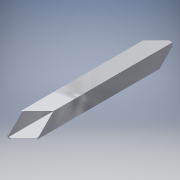
# Autodesk Inventor part: vertical support
Saved by Autodesk Inventor 2016 (Build 200138000, 138)
## iProperties
Created: 2016-02-02
Part Number: vertical support
Material: Aluminum 6061
Document SubType Name: Modeling
Designer: gus
Density: 2.7 g/cm^3
Appearance: Aluminum - Flat
Mass: 93.3295 g
Surface Area: 438.507 cm^2
Volume: 34.5665 cm^3
Author: gus
Autodesk Inventor part; units mm, degrees
ref_plane "YZ Plane" through (0, 0, 0) normal (1, 0, 0) x (0, 1, 0)
ref_plane "XZ Plane" through (0, 0, 0) normal (0, 1, 0) x (-1, 0, 0)
ref_plane "XY Plane" through (0, 0, 0) normal (0, 0, 1) x (1, 0, 0)
sketch "Sketch1" plane through (0, 0, 0) normal (0, 0, 1) x (1, 0, 0)
  line L0 (0, 0) -> (25.4, 0)
  line L1 (25.4, 0) -> (25.4, -25.4)
  line L2 (25.4, -25.4) -> (0, -25.4)
  line L3 (0, -25.4) -> (0, 0)
  line L4 (1.5875, -23.8125) -> (23.8125, -23.8125)
  line L5 (23.8125, -23.8125) -> (23.8125, -1.5875)
  line L6 (23.8125, -1.5875) -> (1.5875, -1.5875)
  line L7 (1.5875, -1.5875) -> (1.5875, -23.8125)
  dimension "d0" = 25.4
  dimension "d1" = 25.4
  dimension "d2" = 1.5875
  constraints: 16 end point, 4 parallel, 2 perpendicular, 1 horizontal, 3 other
  measures "d0" distance of L1.end L2.end
  measures "d1" distance of L0.end L1.end
  measures "d2" distance between parallel lines of L2 L4
extrude "Extrusion1" add sketch "Sketch1" along normal blind 127
sketch "Sketch2" plane through (25.4, -25.4, 0) normal (1, 0, 0) x (0, 0, -1)
  circle A0 centre (-12.7, 12.7) radius 3.3734
  circle A1 centre (-38.1, 12.7) radius 3.3734
  circle A2 centre (-88.9, 12.7) radius 3.3734
  circle A3 centre (-114.3, 12.7) radius 3.3734
  line L0 (0, 25.4) -> (0, 0) projected
  line L1 (0, 25.4) -> (-127, 25.4) projected
  line L2 (0, 0) -> (-127, 0) projected
  line L3 (-127, 0) -> (-127, 25.4) projected
  dimension "d5" = 6.7469
  dimension "d7" = 12.7
  dimension "d8" = 12.7
  dimension "d9" = 12.7
  dimension "d10" = 38.1
  dimension "d11" = 12.7
  dimension "d12" = 38.1
  dimension "d13" = 12.7
  dimension "d14" = 12.7
  constraints: 4 centre point, 3 equal radius
  measures "d5" diameter of A0
  measures "d7" distance from line of A0.centre L0
  measures "d8" distance from line of L1 A0.centre
  measures "d9" distance from line of L2 A1.centre
  measures "d10" distance from line of L0 A1.centre
  measures "d11" distance from line of L3 A3.centre
  measures "d12" distance from line of L3 A2.centre
  measures "d13" distance from line of L2 A2.centre
  measures "d14" distance from line of L2 A3.centre
extrude "Extrusion2" cut sketch "Sketch2" against normal blind 25.4 contours A0 | A1 | A2 | A3
body "Solid1"
